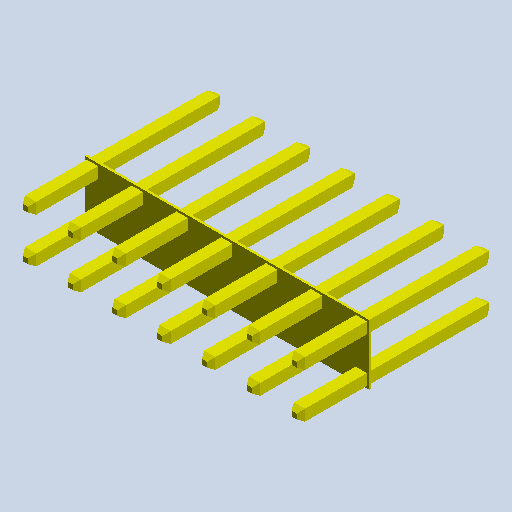
# Autodesk Inventor part: T-1S6-07-TSW-1-07-7-D
Saved by Autodesk Inventor 2024.2 (Build 282272000, 272)
## iProperties
Category: PARTsolutions
Company: SAMTEC
Part Number: T-1S6-07-TSW-1-07-7-D
Material: Generic
Catalog Web Link: www.cadenas.de
Description: TSW Series Pin-TSW Series - (2,54 mm) .100" Through-Hole .025" Square Post Header
Vendor: SAMTEC
Document SubType Name: Modeling
Designer: partserver
Manufacturer: SAMTEC
Mass: 0.0664083 g
Surface Area: 4.8682 cm^2
Volume: 0.0664083 cm^3
Density: 1 g/cm^3
Appearance: PSOLRGB-255-255-0
PSOL_IDENT_0: {$CADENAS_DATA\23d-libs\samtec\modelling\tsw\parts\tsw_pin.prj},222 {VTYP=3D},{NB=T-1S6-07-TSW-1-07-
PSOL_IDENT_1: 7-D},{LINA=T-1S6-07-TSW-1-07-7-D},{NN=TSW Series Pin},{DATE=29.08.2019 09:17:37},{GEOMDATE=10.06.201
PSOL_IDENT_2: 9 10:17:41},{VERSION=},{LINEID=30},{WBVAR=TSS,POS,TOPT,ROW,POLOPT,LLOPT},{WBNUMERIC=POS}  {NB=T-1S6-
PSOL_IDENT_3: 07-TSW-1-07-7-D},{LINA=T-1S6-07-TSW-1-07-7-D},{KT=DUMMY},{PN=T-1S6-07},{TSS=-1},{POS=7},{TOPT=},{TOP
PSOL_IDENT_4: TALG= '','Straight Body' },{ROW=-D},{ROWALG= '-S','-S - Single','-D','-D - Double','-T','-T - Triple'
PSOL_IDENT_5: ,'-Q','-Q - Triple (Fill Outer Rows only)' },{POLOPT=},{POLOPTALG= '','Not Selected','001','001','00
PSOL_IDENT_6: 2','002','003','003','004','004','005','005','006','006','007','007','008','008','009','009','010','
PSOL_IDENT_7: 010','011','011','012','012','013','013','014','014' },{POLOPTMAX=168},{POLOPTMAX2='001','001','002'
PSOL_IDENT_8: ,'002','003','003','004','004','005','005','006','006','007','007','008','008','009','009','010','01
PSOL_IDENT_9: 0','011','011','012','012','013','013','014','014'},{POLARIZE='001','001','002','002','003','003','0
PSOL_IDENT_10: 04','004','005','005','006','006','007','007','008','008','009','009','010','010','011','011','012','
PSOL_IDENT_11: 012','013','013','014','014','015','015','016','016','017','017','018','018','019','019','020','020'
PSOL_IDENT_12: ,'021','021','022','022','023','023','024','024','025','025','026','026','027','027','028','028','02
PSOL_IDENT_13: 9','029','030','030','031','031','032','032','033','033','034','034','035','035','036','036','037','
PSOL_IDENT_14: 037','038','038','039','039','040','040','041','041','042','042','043','043','044','044','045','045'
PSOL_IDENT_15: ,'046','046','047','047','048','048','049','049','050','050','051','051','052','052','053','053','05
PSOL_IDENT_16: 4','054','055','055','056','056','057','057','058','058','059','059','060','060','061','061','062','
PSOL_IDENT_17: 062','063','063','064','064','065','065','066','066','067','067','068','068','069','069','070','070'
PSOL_IDENT_18: ,'071','071','072','072','073','073','074','074','075','075','076','076','077','077','078','078','07
PSOL_IDENT_19: 9','079','080','080','081','081','082','082','083','083','084','084','085','085','086','086','087','
PSOL_IDENT_20: 087','088','088','089','089','090','090','091','091','092','092','093','093','094','094','095','095'
PSOL_IDENT_21: ,'096','096','097','097','098','098','099','099','100','100','101','101','102','102','103','103','10
PSOL_IDENT_22: 4','104','105','105','106','106','107','107','108','108','109','109','110','110','111','111','112','
PSOL_IDENT_23: 112','113','113','114','114','115','115','116','116','117','117','118','118','119','119','120','120'
PSOL_IDENT_24: ,'121','121','122','122','123','123','124','124','125','125','126','126','127','127','128','128','12
PSOL_IDENT_25: 9','129','130','130','131','131','132','132','133','133','134','134','135','135','136','136','137','
PSOL_IDENT_26: 137','138','138','139','139','140','140','141','141','142','142','143','143','144','144','145','145'
PSOL_IDENT_27: ,'146','146','147','147','148','148','149','149','150','150'},{POLOPTATOF=0},{POLOPTPN=},{LLOPT=},{L
PSOL_IDENT_28: LOPTALG= '','Not Selected','-LL','-LL - Locking Lead' },{POLOE=0},{LS=-07},{AS=0.100},{BS=0.430},{CS=
PSOL_IDENT_29: 0.230},{ARA=0.000},{ARE=0.000},{ANA=0.000},{ANE=0.000},{BRANA=0.000},{BRENE=0.000},{CRANA=0.000},{CR
PSOL_IDENT_30: ENE=0.000},{BW=0.20000},{PM=1.00000},{PP=-0.06250},{A=0.70000},{POLPX=-0.2875},{POLPY=0.0000},{POL3D
PSOL_IDENT_31: B=0},{POSOE=1},{LLP=0.000},{D=0.160},{ST= '','Straight Body' },{RA=},{RE=},{NA=},{NE=},{LA=},{AP=0.1
PSOL_IDENT_32: 00},{BP=0.43},{CP=0.230},{BW2=0.160}
NB: T-1S6-07-TSW-1-07-7-D
NN: TSW Series Pin
NT: TSW Series - (2,54 mm) .100" Through-Hole .025" Square Post Header
NBSYN: $PN.-TSW$TSS.$LS.-$POS.$TOPT.$ROW.$POLOPTPN.$LLOPT.
LINA: T-1S6-07-TSW-1-07-7-D
CATALOG: Samtec
PN: T-1S6-07
TSS: -1 - .100 [2.54] Fill every position
POS: 7
TOPT: Straight Body
ROW: -D - Double
POLOPT: Not Selected
LLOPT: Not Selected
LS: -07
AS: 0.1
BS: 0.43
CS: 0.23
ARA: 0
ARE: 0
ANA: 0
ANE: 0
BRANA: 0
BRENE: 0
CRANA: 0
CRENE: 0
SUPPLIER: SAMTEC
ARTICLENO: T-1S6-07-TSW-1-07-7-D
BOMINFO: T-1S6-07-TSW-1-07-7-D
CREATOR: CADENAS GmbH
Title: T-1S6-07-TSW-1-07-7-D
Author: Cadenas PARTsolutions
Comments: TSW Series - (2,54 mm) .100" Through-Hole .025" Square Post Header
Autodesk Inventor part; units mm, degrees
sketch "Sketch_1" plane through (0, 0, 0) normal (0, 0, 1) x (1, 0, 0)
  line L0 (-7.9375, 10.922) -> (-7.9375, 0)
  line L1 (-7.9375, 0) -> (7.9375, 0)
  line L2 (7.9375, 0) -> (7.9375, 10.922)
  line L3 (7.9375, 10.922) -> (-7.9375, 10.922)
  constraints: 8 end point
extrude "Extrusion1" add sketch "Sketch_1" along normal mid plane 3.175
sketch "Sketch_26" plane through (0, 0, 0) normal (1, 0, 0) x (0, 1, 0)
  line L0 (3.937, 1.7145) -> (3.81, 1.7145)
  line L1 (3.81, 1.7145) -> (3.81, -1.7145)
  line L2 (3.81, -1.7145) -> (3.937, -1.7145)
  line L3 (3.937, -1.7145) -> (3.937, 1.7145)
  constraints: 8 end point
extrude "Extrusion2" add sketch "Sketch_26" along normal mid plane 16.129
sketch "Sketch_9" plane through (0, 0, 0) normal (0, 0, 1) x (1, 0, 0)
  line L0 (-7.3025, 14.859) -> (-7.3025, 3.937)
  line L1 (-7.3025, 3.937) -> (-5.3975, 3.937)
  line L2 (-5.3975, 3.937) -> (-5.3975, 10.922)
  line L3 (-5.3975, 10.922) -> (-4.7625, 10.922)
  line L4 (-4.7625, 10.922) -> (-4.7625, 3.937)
  line L5 (-4.7625, 3.937) -> (-2.8575, 3.937)
  line L6 (-2.8575, 3.937) -> (-2.8575, 10.922)
  line L7 (-2.8575, 10.922) -> (-2.2225, 10.922)
  line L8 (-2.2225, 10.922) -> (-2.2225, 3.937)
  line L9 (-2.2225, 3.937) -> (-0.3175, 3.937)
  line L10 (-0.3175, 3.937) -> (-0.3175, 10.922)
  line L11 (-0.3175, 10.922) -> (0.3175, 10.922)
  line L12 (0.3175, 10.922) -> (0.3175, 3.937)
  line L13 (0.3175, 3.937) -> (2.2225, 3.937)
  line L14 (2.2225, 3.937) -> (2.2225, 10.922)
  line L15 (2.2225, 10.922) -> (2.8575, 10.922)
  line L16 (2.8575, 10.922) -> (2.8575, 3.937)
  line L17 (2.8575, 3.937) -> (4.7625, 3.937)
  line L18 (4.7625, 3.937) -> (4.7625, 10.922)
  line L19 (4.7625, 10.922) -> (5.3975, 10.922)
  line L20 (5.3975, 10.922) -> (5.3975, 3.937)
  line L21 (5.3975, 3.937) -> (7.3025, 3.937)
  line L22 (7.3025, 3.937) -> (7.3025, 14.859)
  line L23 (7.3025, 14.859) -> (-7.3025, 14.859)
  constraints: 48 end point
extrude "Extrusion3" cut sketch "Sketch_9" along normal mid plane 10.16
sketch "Sketch_12" plane through (0, 0, 0) normal (0, 0, 1) x (1, 0, 0)
  line L0 (-7.3025, -7.112) -> (7.3025, -7.112)
  line L1 (7.3025, -7.112) -> (7.3025, 3.81)
  line L2 (7.3025, 3.81) -> (5.3975, 3.81)
  line L3 (5.3975, 3.81) -> (5.3975, 0)
  line L4 (5.3975, 0) -> (4.7625, 0)
  line L5 (4.7625, 0) -> (4.7625, 3.81)
  line L6 (4.7625, 3.81) -> (2.8575, 3.81)
  line L7 (2.8575, 3.81) -> (2.8575, 0)
  line L8 (2.8575, 0) -> (2.2225, 0)
  line L9 (2.2225, 0) -> (2.2225, 3.81)
  line L10 (2.2225, 3.81) -> (0.3175, 3.81)
  line L11 (0.3175, 3.81) -> (0.3175, 0)
  line L12 (0.3175, 0) -> (-0.3175, 0)
  line L13 (-0.3175, 0) -> (-0.3175, 3.81)
  line L14 (-0.3175, 3.81) -> (-2.2225, 3.81)
  line L15 (-2.2225, 3.81) -> (-2.2225, 0)
  line L16 (-2.2225, 0) -> (-2.8575, 0)
  line L17 (-2.8575, 0) -> (-2.8575, 3.81)
  line L18 (-2.8575, 3.81) -> (-4.7625, 3.81)
  line L19 (-4.7625, 3.81) -> (-4.7625, 0)
  line L20 (-4.7625, 0) -> (-5.3975, 0)
  line L21 (-5.3975, 0) -> (-5.3975, 3.81)
  line L22 (-5.3975, 3.81) -> (-7.3025, 3.81)
  line L23 (-7.3025, 3.81) -> (-7.3025, -7.112)
  constraints: 48 end point
extrude "Extrusion4" cut sketch "Sketch_12" along normal mid plane 10.16
sketch "Sketch_14" plane through (0, 0, 0) normal (1, 0, 0) x (0, 1, 0)
  line L0 (14.859, 0.9525) -> (3.937, 0.9525)
  line L1 (3.937, 0.9525) -> (3.937, -0.9525)
  line L2 (3.937, -0.9525) -> (14.859, -0.9525)
  line L3 (14.859, -0.9525) -> (14.859, 0.9525)
  constraints: 8 end point
extrude "Extrusion5" cut sketch "Sketch_14" along normal mid plane 35.56
sketch "Sketch_16" plane through (0, 0, 0) normal (1, 0, 0) x (0, 1, 0)
  line L0 (-7.112, 0.9525) -> (-7.112, -0.9525)
  line L1 (-7.112, -0.9525) -> (3.81, -0.9525)
  line L2 (3.81, -0.9525) -> (3.81, 0.9525)
  line L3 (3.81, 0.9525) -> (-7.112, 0.9525)
  constraints: 8 end point
extrude "Extrusion6" cut sketch "Sketch_16" along normal mid plane 35.56
sketch "Sketch_40" plane through (0, 0, 0) normal (1, 0, 0) x (0, 1, 0)
  line L0 (10.6172, 1.5875) -> (10.922, 1.4115)
  line L1 (10.922, 1.4115) -> (10.922, 1.1285)
  line L2 (10.922, 1.1285) -> (10.6172, 0.9525)
  line L3 (10.6172, 0.9525) -> (10.6172, -0.9525)
  line L4 (10.6172, -0.9525) -> (10.922, -1.1285)
  line L5 (10.922, -1.1285) -> (10.922, -1.4115)
  line L6 (10.922, -1.4115) -> (10.6172, -1.5875)
  line L7 (10.6172, -1.5875) -> (13.1572, -1.5875)
  line L8 (13.1572, -1.5875) -> (13.1572, 1.5875)
  line L9 (13.1572, 1.5875) -> (10.6172, 1.5875)
  constraints: 20 end point
extrude "Extrusion7" cut sketch "Sketch_40" along normal mid plane 35.56
sketch "Sketch_44" plane through (0, 0, 0) normal (1, 0, 0) x (0, 1, 0)
  line L0 (0.3048, 1.5875) -> (-2.2352, 1.5875)
  line L1 (-2.2352, 1.5875) -> (-2.2352, -1.5875)
  line L2 (-2.2352, -1.5875) -> (0.3048, -1.5875)
  line L3 (0.3048, -1.5875) -> (0, -1.4115)
  line L4 (0, -1.4115) -> (0, -1.1285)
  line L5 (0, -1.1285) -> (0.3048, -0.9525)
  line L6 (0.3048, -0.9525) -> (0.3048, 0.9525)
  line L7 (0.3048, 0.9525) -> (0, 1.1285)
  line L8 (0, 1.1285) -> (0, 1.4115)
  line L9 (0, 1.4115) -> (0.3048, 1.5875)
  constraints: 20 end point
extrude "Extrusion8" cut sketch "Sketch_44" along normal mid plane 35.56
sketch "Sketch_45" plane through (0, 0, 0) normal (0, 0, 1) x (1, 0, 0)
  line L0 (-7.9375, 10.6172) -> (-7.7615, 10.922)
  line L1 (-7.7615, 10.922) -> (-7.4785, 10.922)
  line L2 (-7.4785, 10.922) -> (-7.3025, 10.6172)
  line L3 (-7.3025, 10.6172) -> (-5.3975, 10.6172)
  line L4 (-5.3975, 10.6172) -> (-5.2215, 10.922)
  line L5 (-5.2215, 10.922) -> (-4.9385, 10.922)
  line L6 (-4.9385, 10.922) -> (-4.7625, 10.6172)
  line L7 (-4.7625, 10.6172) -> (-2.8575, 10.6172)
  line L8 (-2.8575, 10.6172) -> (-2.6815, 10.922)
  line L9 (-2.6815, 10.922) -> (-2.3985, 10.922)
  line L10 (-2.3985, 10.922) -> (-2.2225, 10.6172)
  line L11 (-2.2225, 10.6172) -> (-0.3175, 10.6172)
  line L12 (-0.3175, 10.6172) -> (-0.1415, 10.922)
  line L13 (-0.1415, 10.922) -> (0.1415, 10.922)
  line L14 (0.1415, 10.922) -> (0.3175, 10.6172)
  line L15 (0.3175, 10.6172) -> (2.2225, 10.6172)
  line L16 (2.2225, 10.6172) -> (2.3985, 10.922)
  line L17 (2.3985, 10.922) -> (2.6815, 10.922)
  line L18 (2.6815, 10.922) -> (2.8575, 10.6172)
  line L19 (2.8575, 10.6172) -> (4.7625, 10.6172)
  line L20 (4.7625, 10.6172) -> (4.9385, 10.922)
  line L21 (4.9385, 10.922) -> (5.2215, 10.922)
  line L22 (5.2215, 10.922) -> (5.3975, 10.6172)
  line L23 (5.3975, 10.6172) -> (7.3025, 10.6172)
  line L24 (7.3025, 10.6172) -> (7.4785, 10.922)
  line L25 (7.4785, 10.922) -> (7.7615, 10.922)
  line L26 (7.7615, 10.922) -> (7.9375, 10.6172)
  line L27 (7.9375, 10.6172) -> (7.9375, 13.1572)
  line L28 (7.9375, 13.1572) -> (-7.9375, 13.1572)
  line L29 (-7.9375, 13.1572) -> (-7.9375, 10.6172)
  constraints: 60 end point
extrude "Extrusion9" cut sketch "Sketch_45" along normal mid plane 10.16
sketch "Sketch_46" plane through (0, 0, 0) normal (0, 0, 1) x (1, 0, 0)
  line L0 (-7.9375, 0.3048) -> (-7.9375, -2.2352)
  line L1 (-7.9375, -2.2352) -> (7.9375, -2.2352)
  line L2 (7.9375, -2.2352) -> (7.9375, 0.3048)
  line L3 (7.9375, 0.3048) -> (7.7615, 0)
  line L4 (7.7615, 0) -> (7.4785, 0)
  line L5 (7.4785, 0) -> (7.3025, 0.3048)
  line L6 (7.3025, 0.3048) -> (5.3975, 0.3048)
  line L7 (5.3975, 0.3048) -> (5.2215, 0)
  line L8 (5.2215, 0) -> (4.9385, 0)
  line L9 (4.9385, 0) -> (4.7625, 0.3048)
  line L10 (4.7625, 0.3048) -> (2.8575, 0.3048)
  line L11 (2.8575, 0.3048) -> (2.6815, 0)
  line L12 (2.6815, 0) -> (2.3985, 0)
  line L13 (2.3985, 0) -> (2.2225, 0.3048)
  line L14 (2.2225, 0.3048) -> (0.3175, 0.3048)
  line L15 (0.3175, 0.3048) -> (0.1415, 0)
  line L16 (0.1415, 0) -> (-0.1415, 0)
  line L17 (-0.1415, 0) -> (-0.3175, 0.3048)
  line L18 (-0.3175, 0.3048) -> (-2.2225, 0.3048)
  line L19 (-2.2225, 0.3048) -> (-2.3985, 0)
  line L20 (-2.3985, 0) -> (-2.6815, 0)
  line L21 (-2.6815, 0) -> (-2.8575, 0.3048)
  line L22 (-2.8575, 0.3048) -> (-4.7625, 0.3048)
  line L23 (-4.7625, 0.3048) -> (-4.9385, 0)
  line L24 (-4.9385, 0) -> (-5.2215, 0)
  line L25 (-5.2215, 0) -> (-5.3975, 0.3048)
  line L26 (-5.3975, 0.3048) -> (-7.3025, 0.3048)
  line L27 (-7.3025, 0.3048) -> (-7.4785, 0)
  line L28 (-7.4785, 0) -> (-7.7615, 0)
  line L29 (-7.7615, 0) -> (-7.9375, 0.3048)
  constraints: 60 end point
extrude "Extrusion10" cut sketch "Sketch_46" along normal mid plane 10.16
ref_plane "pin_XY" through (0, 2.54, 0) normal (0, 1, 0) x (1, 0, 0)
ref_plane "pin_YZ" through (0, 2.54, 0) normal (1, 0, 0) x (0, 0, -1)
ref_plane "pin_ZX" through (0, 2.54, 0) normal (0, 0, -1) x (0, 1, 0)
ref_plane "zst_prj_pin_XY" through (0, 0, 0) normal (0, 1, 0) x (1, 0, 0)
ref_plane "zst_prj_pin_YZ" through (0, 0, 0) normal (1, 0, 0) x (0, 0, -1)
ref_plane "zst_prj_pin_ZX" through (0, 0, 0) normal (0, 0, -1) x (0, 1, 0)
body "Solid1"
